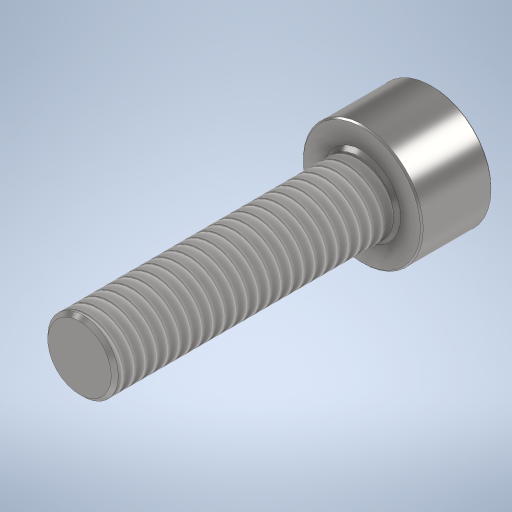
# Autodesk Inventor part: SHCSM5x20
Saved by Autodesk Inventor 2024 (Build 280153000, 153)
## iProperties
Created: 2024-09-05
Part Number: SHCSM5x20
Material: Stainless Steel
Document SubType Name: Modeling
Designer: Ishaan
Density: 8 g/cm^3
Appearance: Semi-Polished
Author: Ishaan
Autodesk Inventor part; units mm, degrees
ref_plane "YZ Plane" through (0, 0, 0) normal (1, 0, 0) x (0, 1, 0)
ref_plane "XZ Plane" through (0, 0, 0) normal (0, 1, 0) x (-1, 0, 0)
ref_plane "XY Plane" through (0, 0, 0) normal (0, 0, 1) x (1, 0, 0)
sketch "Sketch1" plane through (0, 0, 0) normal (0, 0, 1) x (1, 0, 0)
  circle A0 centre (0, 0) radius 4.25
  circle A1 centre (0, 0) radius 2.5
  dimension "d0" = 8.5
  dimension "d1" = 5
  constraints: 2 centre point, 2 coincident
  measures "d0" diameter of A0
  measures "d1" diameter of A1
extrude "Extrusion1" add sketch "Sketch1" along normal blind 20 contours A1
extrude "Extrusion2" add sketch "Sketch1" against normal blind 5 contours A0 | A1
thread "Thread1" size "M5x0.8" class "6g" standard "ANSI Metric M Profile" full length
chamfer "Chamfer1" distance 0.1 angle 45 2 edges at (-4.25, 0, 0) (-4.25, 0, -5)
sketch "Sketch2" plane through (0, 0, -5) normal (0, 0, -1) x (-1, 0, 0)
  circle A0 centre (0, 0) radius 1.875
  line L0 (-1.1547, 2) -> (1.1547, 2)
  line L1 (1.1547, 2) -> (2.3094, 0)
  line L2 (2.3094, 0) -> (1.1547, -2)
  line L3 (1.1547, -2) -> (-1.1547, -2)
  line L4 (-1.1547, -2) -> (-2.3094, 0)
  line L5 (-2.3094, 0) -> (-1.1547, 2)
  dimension "d11" = 3.75
  dimension "d12" = 4
  constraints: 12 end point, 2 coincident, 1 centre point, 1 horizontal, 13 other
  measures "d11" diameter of A0
  measures "d12" distance between parallel lines of L3 L0
hole "Hole1" at (0, 0, -5) direction (0, 0, 1) diameter 3.75 depth 2.5 tip angle 150
chamfer "Chamfer2" distance 0.5 angle 45 1 edges at (0, -1.875, -5)
extrude "Extrusion4" cut sketch "Sketch2" against normal up to surface contours A0 | L0 L1 L2 L3 L4 L5 round surface about axis through (0, 0, -2.2488) along (0, 0, -1) radius 0.9375 half angle 75 far side no
chamfer "Chamfer3" distance 0.25 angle 45 2 edges at (-2.5, 0, 0) (-2.5, 0, 20)
equation "\"d23\" = d11"
body "Solid1"
